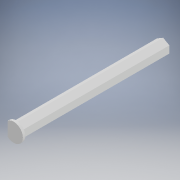
# Autodesk Inventor part: Fake Hex Rod 6in
Saved by Autodesk Inventor 2020 (Build 240168000, 168)
## iProperties
Created: 2021-03-29
Part Number: Fake Hex Rod 6in
Material: Generic
Document SubType Name: Modeling
Designer: sidsa
Density: 1 g/cm^3
Appearance: Default
Author: sidsa
## iProperties of the stored document _3DPrint.ipt
Created: 2021-03-29
Part Number: _3DPrint
Material: Generic
Document SubType Name: Modeling
Designer: sidsa
Density: 1 g/cm^3
Appearance: Default
Author: sidsa
Autodesk Inventor part; units mm, degrees
ref_plane "YZ Plane" through (0, 0, 0) normal (1, 0, 0) x (0, 1, 0)
ref_plane "XZ Plane" through (0, 0, 0) normal (0, 1, 0) x (-1, 0, 0)
ref_plane "XY Plane" through (0, 0, 0) normal (0, 0, 1) x (1, 0, 0)
sketch "Sketch1" plane through (0, 0, 0) normal (0, 0, 1) x (1, 0, 0)
  line L0 (0, 7.3323) -> (6.35, 3.6662)
  line L1 (6.35, 3.6662) -> (6.35, -3.6662)
  line L2 (6.35, -3.6662) -> (0, -7.3323)
  line L3 (0, -7.3323) -> (-6.35, -3.6662)
  line L4 (-6.35, -3.6662) -> (-6.35, 3.6662)
  line L5 (-6.35, 3.6662) -> (0, 7.3323)
  point P0 (0, 0)
  point P1 (0, 0)
  dimension "d0" = 12.7
  constraints: 12 end point, 1 coincident, 13 other
  measures "d0" distance between parallel lines of L1 L4
extrude "Extrusion1" add sketch "Sketch1" along normal blind 152.4
sketch "Sketch2" plane through (0, 0, 152.4) normal (0, 0, 1) x (1, 0, 0)
  circle A0 centre (0, 0) radius 9.525
  line L0 (-6.35, 3.6662) -> (-6.35, -3.6662) projected
  line L1 (6.35, 3.6662) -> (0, 7.3323) projected
  line L2 (0, 7.3323) -> (-6.35, 3.6662) projected
  line L3 (-6.35, 3.6662) -> (-6.35, -3.6662) projected
  line L4 (-6.35, -3.6662) -> (0, -7.3323) projected
  line L5 (0, -7.3323) -> (6.35, -3.6662) projected
  line L6 (6.35, -3.6662) -> (6.35, 3.6662) projected
  line L7 (-6.35, 3.6662) -> (-6.35, 7.0995)
  line L8 (-6.35, -3.6662) -> (-6.35, -7.0995)
  point P0 (-6.35, -3.6662)
  dimension "d3" = 19.05
  constraints: 4 end point, 2 point on circle, 1 centre point, 1 coincident, 1 point on line, 1 vertical
  measures "d3" diameter of A0
extrude "Extrusion2" add sketch "Sketch2" along normal blind 2.54 contours A0 L8 L4 L5 L6 L1 L2 L7 | L2 L1 L6 L5 L4 L0
body "Solid1"
